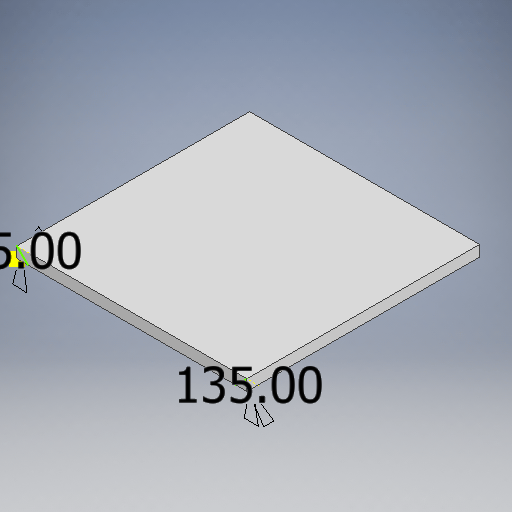
# Autodesk Inventor part: 1ipt
Saved by Autodesk Inventor 2025.2 (Build 292293000, 293)
## iProperties
Created: 2025-03-17
Part Number: 1ipt
Material: 일반
Document SubType Name: Modeling
Designer: jbhma
Density: 1 g/cm^3
Appearance: 기본값
Author: jbhma
Autodesk Inventor part; units mm, degrees
ref_plane "YZ Plane" through (0, 0, 0) normal (1, 0, 0) x (0, 1, 0)
ref_plane "XZ Plane" through (0, 0, 0) normal (0, 1, 0) x (-1, 0, 0)
ref_plane "XY Plane" through (0, 0, 0) normal (0, 0, 1) x (1, 0, 0)
sketch "스케치1" plane through (0, 0, 0) normal (0, 1, 0) x (-1, 0, 0)
  line L0 (0, 0) -> (-420, 0)
  line L1 (-420, 0) -> (-420, -425)
  line L2 (-420, -425) -> (0, -425)
  line L3 (0, -425) -> (0, 0)
  dimension "d0" = 420
  dimension "d1" = 425
  constraints: 8 end point, 2 parallel, 1 horizontal, 1 perpendicular
  measures "d0" distance of L2.end L1.end
  measures "d1" distance of L1.end L0.end
extrude "돌출1" add sketch "스케치1" along normal blind 20
sketch "스케치2" plane through (0, 0, 0) normal (0, 0, 1) x (1, 0, 0)
  line L0 (0, 20) -> (20, 0)
  line L1 (0, 20) -> (28.2843, 20) construction
  line L2 (420, 20) -> (442.6274, 20) construction
  line L3 (420, 20) -> (400, 0)
  line L4 (420, 20) -> (448.2843, 20) construction
  point P0 (0, 0)
  dimension "d4" = 45
  dimension "d8" = 135
  constraints: 10 end point, 3 horizontal, 2 equal length
  measures "d4" angle of L0 L1
  measures "d8" angle of L3 L4
